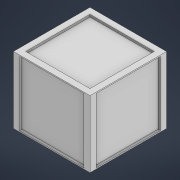
# Autodesk Inventor part: End-Effector
Saved by Autodesk Inventor 2022 (Build 260153000, 153)
## iProperties
Created: 2023-04-20
Part Number: End-Effector
Material: Generic
Document SubType Name: Modeling
Designer: Karl
Density: 1 g/cm^3
Appearance: Default
Author: Karl
Autodesk Inventor part; units mm, degrees
ref_plane "YZ Plane" through (0, 0, 0) normal (1, 0, 0) x (0, 1, 0)
ref_plane "XZ Plane" through (0, 0, 0) normal (0, 1, 0) x (-1, 0, 0)
ref_plane "XY Plane" through (0, 0, 0) normal (0, 0, 1) x (1, 0, 0)
sketch "Sketch3" plane through (0, 0, 0) normal (0, 0, 1) x (1, 0, 0)
  line L0 (0, 0) -> (-55.38, 0)
  line L1 (-55.38, 0) -> (-55.38, 47.03)
  line L2 (-55.38, 47.03) -> (0, 47.03)
  line L3 (0, 47.03) -> (0, 0)
  line L4 (5, -5) -> (5, 52.03)
  line L5 (5, 52.03) -> (-60.38, 52.03)
  line L6 (5, -5) -> (-60.38, -5)
  line L7 (-60.38, -5) -> (-60.38, 52.03)
  dimension "d26" = 47.03
  dimension "d27" = 55.38
  constraints: 16 end point, 3 perpendicular, 2 horizontal, 2 parallel, 1 vertical
  measures "d26" distance of L2.end L0.start
  measures "d27" distance of L0.start L0.end
extrude "Extrusion10" add sketch "Sketch3" along normal blind 60.31
sketch "Sketch12" plane through (0, 0, 60.31) normal (0, 0, 1) x (1, 0, 0)
  line L0 (5, -5) -> (5, 52.03) projected
  line L1 (-60.38, 52.03) -> (-60.38, -5) projected
  line L2 (5, -5) -> (-60.38, -5)
  line L3 (-60.38, -5) -> (-60.38, 52.03)
  line L4 (-60.38, 52.03) -> (5, 52.03)
  line L5 (5, 52.03) -> (5, -5)
  point P0 (0, 0)
  constraints: 8 end point, 2 parallel, 1 horizontal, 1 perpendicular
extrude "Extrusion13" add sketch "Sketch12" along normal blind 5
sketch "Sketch13" plane through (0, 0, 65.31) normal (0, 0, 1) x (1, 0, 0)
  line L0 (5, -5) -> (5, 52.03) projected
  line L1 (5, -5) -> (10.19, -5) construction
  line L2 (-60.38, -5) -> (5, -5) projected
  line L3 (-0.19, -5) -> (0.825, -5) construction
  line L4 (-0.19, -3.985) -> (-55.19, -3.985)
  line L5 (-55.19, -3.985) -> (-55.19, 51.015)
  line L6 (-55.19, 51.015) -> (-0.19, 51.015)
  line L7 (-0.19, 51.015) -> (-0.19, -3.985)
  point P0 (0, 0)
  dimension "d86" = 5.19
  dimension "d88" = 1.015
  dimension "d90" = 55
  dimension "d91" = 55
  constraints: 12 end point, 3 horizontal, 2 parallel, 1 perpendicular
  measures "d86" distance of L0.start L3.start
  measures "d88" distance of L3.start L4.start
  measures "d90" distance of L5.end L6.end
  measures "d91" distance of L4.end L5.end
extrude "Extrusion14" cut sketch "Sketch13" against normal blind 2
sketch "Sketch14" plane through (-60.38, 52.03, 0) normal (0, 1, 0) x (1, 0, 0)
  line L0 (0, -65.31) -> (65.38, -65.31) projected
  line L1 (65.38, -65.31) -> (60.19, -65.31)
  line L2 (65.38, -65.31) -> (70.57, -65.31) construction
  line L3 (60.19, -65.31) -> (60.19, -60.155)
  line L4 (60.19, -65.31) -> (65.345, -65.31) construction
  line L5 (60.19, -60.155) -> (5.19, -60.155)
  line L6 (5.19, -60.155) -> (5.19, -5.155)
  line L7 (5.19, -5.155) -> (60.19, -5.155)
  line L8 (60.19, -5.155) -> (60.19, -60.155)
  point P0 (60.38, 0)
  dimension "d94" = 5.19
  dimension "d95" = 180
  dimension "d96" = 5.155
  dimension "d97" = 90
  dimension "d98" = 55
  dimension "d99" = 55
  constraints: 16 end point, 3 horizontal, 2 equal length, 2 parallel, 1 collinear, 1 perpendicular, 1 vertical
  measures "d94" distance of L0.end L1.end
  measures "d95" angle of L1 L2
  measures "d96" distance of L1.end L3.end
  measures "d97" angle of L4 L3
  measures "d98" distance of L6.end L7.end
  measures "d99" distance of L5.end L6.end
extrude "Extrusion15" cut sketch "Sketch14" against normal blind 2
sketch "Sketch15" plane through (-60.38, -5, 0) normal (0, -1, 0) x (1, 0, 0)
  line L0 (0, 65.31) -> (5.19, 65.31)
  line L1 (65.38, 65.31) -> (0, 65.31) projected
  line L2 (60.19, 60.155) -> (5.19, 60.155) projected
  line L3 (5.19, 65.31) -> (5.19, 60.155)
  line L4 (5.19, 60.155) -> (60.19, 60.155)
  line L5 (60.19, 60.155) -> (60.19, 5.155)
  line L6 (60.19, 5.155) -> (5.19, 5.155)
  line L7 (5.19, 5.155) -> (5.19, 60.155)
  point P0 (60.38, 0)
  dimension "d104" = 5.19
  dimension "d105" = 5.155
  dimension "d106" = 90
  dimension "d107" = 55
  dimension "d108" = 55
  constraints: 12 end point, 2 parallel, 1 horizontal, 1 perpendicular, 1 point on line
  measures "d104" distance of L0.start L0.end
  measures "d105" distance of L0.end L2.end
  measures "d106" angle of L0 L3
  measures "d107" distance of L5.end L6.end
  measures "d108" distance of L4.end L5.end
extrude "Extrusion16" cut sketch "Sketch15" against normal blind 2
sketch "Sketch16" plane through (-60.38, -5, 0) normal (-1, 0, 0) x (0, 0, 1)
  line L0 (0, 57.03) -> (5.155, 57.03)
  line L1 (0, 57.03) -> (5.155, 57.03) construction
  line L2 (5.155, 57.03) -> (5.155, 56.015)
  line L3 (5.155, 56.015) -> (60.155, 56.015)
  line L4 (60.155, 56.015) -> (60.155, 1.015)
  line L5 (60.155, 1.015) -> (5.155, 1.015)
  line L6 (5.155, 1.015) -> (5.155, 56.015)
  point P0 (0, 5)
  dimension "d111" = 5.155
  dimension "d112" = 0
  dimension "d113" = 1.015
  dimension "d114" = 90
  dimension "d115" = 55
  dimension "d116" = 55
  constraints: 14 end point, 2 horizontal, 2 parallel, 2 perpendicular, 1 collinear
  measures "d111" distance of L0.start L0.end
  measures "d112" distance between parallel lines of L0 L1
  measures "d113" distance of L0.end L2.end
  measures "d114" angle of L0 L2
  measures "d115" distance of L4.end L5.end
  measures "d116" distance of L3.end L4.end
extrude "Extrusion17" cut sketch "Sketch16" against normal blind 2
sketch "Sketch17" plane through (5, -5, 0) normal (1, 0, 0) x (0, 0, -1)
  line L0 (0, 57.03) -> (-65.31, 57.03) projected
  line L1 (-65.31, 57.03) -> (-60.155, 57.03)
  line L2 (-65.31, 57.03) -> (-60.155, 57.03) construction
  line L3 (-60.155, 57.03) -> (-60.155, 56.015)
  line L4 (-60.155, 57.03) -> (-59.14, 57.03) construction
  line L5 (-60.155, 56.015) -> (-5.155, 56.015)
  line L6 (-5.155, 56.015) -> (-5.155, 1.015)
  line L7 (-5.155, 1.015) -> (-60.155, 1.015)
  line L8 (-60.155, 1.015) -> (-60.155, 56.015)
  point P0 (0, 5)
  dimension "d119" = 5.155
  dimension "d120" = 0
  dimension "d121" = 1.015
  dimension "d122" = 90
  dimension "d123" = 55
  dimension "d124" = 55
  constraints: 16 end point, 3 horizontal, 2 equal length, 2 parallel, 1 collinear, 1 perpendicular, 1 vertical
  measures "d119" distance of L0.end L1.end
  measures "d120" distance between parallel lines of L1 L2
  measures "d121" distance of L2.end L3.end
  measures "d122" angle of L3 L4
  measures "d123" distance of L6.end L7.end
  measures "d124" distance of L5.end L6.end
extrude "Extrusion18" cut sketch "Sketch17" against normal blind 2
body "Solid3"
